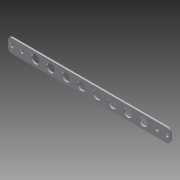
# Autodesk Inventor part: V5 Shooter Frame Channel P7
Saved by Autodesk Inventor 2014 SP1 (Build 180222100, 222)
## iProperties
Created: 2012-02-04
Part Number: V5 Shooter Frame Channel P7
Material: Aluminum-6061
Document SubType Name: Sheet Metal
Designer: Moses
Mass: 49.3461 g
Surface Area: 154.011 cm^2
Volume: 18.2089 cm^3
Density: 2.71 g/cm^3
Sheet Metal Rule: Default
Flat Pattern Width: 2.54 cm
Flat Pattern Length: 30.4548 cm
Flat Pattern Area: 77.3552 cm^2
Sheet Metal Width: 1.000 in
Sheet Metal Length: 11.990 in
Sheet Metal Area: 11.990 in^2
Appearance: Aluminum - Flat
Author: Moses
Autodesk Inventor part; units mm, degrees
ref_plane "YZ Plane" through (0, 0, 0) normal (1, 0, 0) x (0, 1, 0)
ref_plane "XZ Plane" through (0, 0, 0) normal (0, 1, 0) x (-1, 0, 0)
ref_plane "XY Plane" through (0, 0, 0) normal (0, 0, 1) x (1, 0, 0)
sketch "Sketch1" plane through (0, 0, 0) normal (0, 0, 1) x (1, 0, 0)
  arc A0 (-9.525, 55.0553) -> (-15.875, 48.7053) centre (-9.525, 48.7053) ccw construction
  line L0 (-15.875, 19.05) -> (-15.875, 48.7053) construction
  line L1 (-15.875, 19.05) -> (15.875, 19.05) construction
  line L2 (15.875, 48.7053) -> (15.875, 19.05) construction
  arc A1 (15.875, 48.7053) -> (9.525, 55.0553) centre (9.525, 48.7053) ccw construction
  line L3 (-9.525, 55.0553) -> (9.525, 55.0553) construction
  circle A2 centre (9.525, 42.3553) radius 3.3782 projected
  circle A3 centre (-9.525, 42.3553) radius 3.3782 projected
  arc A4 (-256.923, 48.7053) -> (-263.273, 55.0553) centre (-263.273, 48.7053) ccw construction
  line L4 (-282.323, 55.0553) -> (-263.273, 55.0553) construction
  arc A5 (-282.323, 55.0553) -> (-288.673, 48.7053) centre (-282.323, 48.7053) ccw construction
  line L5 (-288.673, 19.05) -> (-288.673, 48.7053) construction
  line L6 (-288.673, 19.05) -> (-256.923, 19.05) construction
  line L7 (-256.923, 48.7053) -> (-256.923, 19.05) construction
  circle A6 centre (-263.273, 42.3553) radius 3.3782 projected
  circle A7 centre (-282.323, 42.3553) radius 3.3782 projected
  line L8 (-288.673, 55.0553) -> (15.875, 55.0553)
  line L9 (-288.673, 29.6553) -> (15.875, 29.6553)
  line L10 (-288.673, 29.6553) -> (-288.673, 55.0553)
  line L11 (15.875, 29.6553) -> (15.875, 55.0553)
  line L12 (-288.673, 42.3553) -> (15.875, 42.3553) construction
  circle A8 centre (-237.873, 42.3553) radius 7.9375
  circle A9 centre (-208.8804, 42.3553) radius 7.9375
  circle A10 centre (-179.8879, 42.3553) radius 7.9375
  circle A11 centre (-150.8953, 42.3553) radius 7.9375
  circle A12 centre (-121.9027, 42.3553) radius 7.9375
  circle A13 centre (-92.9101, 42.3553) radius 7.9375
  circle A14 centre (-63.9176, 42.3553) radius 7.9375
  circle A15 centre (-34.925, 42.3553) radius 7.9375
  point P0 (0, 0)
  dimension "d1" = 25.4
  dimension "d2" = 12.7
  dimension "d33" = 15.875
  dimension "d35" = 304.548
  dimension "d36" = 50.8
  dimension "d39" = 28.9926
  constraints: 10 end point, 8 centre point, 3 parallel, 3 point on line, 2 midpoint, 2 perpendicular, 1 horizontal, 14 other
  measures "d1" distance between parallel lines of L8 L9
  measures "d2" distance from line of L8 A7.centre
  measures "d33" diameter of A8
  measures "d35" distance of L12.start L12.end
  measures "d36" distance from line of L5 A8.centre
  measures "d39" distance of A8.centre A9.centre
extrude "Plate1" add sketch "Sketch1" along normal blind 3.048
fillet "Corner Round1" radius 6.35 4 edges at (-288.673, 29.6553, 1.524) (-288.673, 55.0553, 1.524) (15.875, 29.6553, 1.524) (15.875, 55.0553, 1.524)
equation "\"d39\" = -0.285714 * d36 + 0.142857 * d35"
equation "\"BendRadius\" = Thickness"
equation "\"BendReliefWidth\" = Thickness"
equation "\"BendReliefDepth\" = 0.5 * Thickness"
equation "\"CornerReliefSize\" = 4 * Thickness"
equation "\"MinimumRemnant\" = 2 * Thickness"
equation "\"TransitionRadius\" = BendRadius"
equation "\"JacobiRadiusSize\" = BendRadius"
equation "\"GapSize\" = Thickness"
equation "\"d3\" = BendRadius"
equation "\"Thickness\" = 3.048"
body "Solid1"
